Autodesk Fusion 360 part; units mm, degrees
(part 9 of 9)
extrude "Extrude4''" add sketch "Sketch1 (3)" along normal blind 2 contours A4 L3 A7 L4 L6 | A4 L2 A7 L5 L7 | A4 A5 L6 L7 | A7 A8 L6 L7 picked at (-8.5623, -94.7426) picked at (8.642, -94.7512) picked at (-12.4732, -65.0425) picked at (-12.3684, -117.2548) bodies 6 in component "Base"
extrude "Extrude5'" add sketch "Sketch1 (3)" along normal blind 1 from surface at 2 contours A4 A5 L6 L8 | A4 A7 L6 L8 | A7 A8 L6 L8 | A4 A7 L7 L9 | A4 A5 L7 L9 | A7 A8 L7 L9 | A5 L7 A9 L8 L9 | A8 A10 L8 L9 picked at (-4.204, -76.7531) picked at (-3.6307, -94.1364) picked at (-4.18, -104.3491) picked at (3.6752, -86.9585) picked at (4.2245, -76.7458) picked at (4.2486, -104.3417) picked at (-4.5123, -61.3284) picked at (5.702, -117.4496) bodies 6 7 in component "Base"
extrude "Extrude6" add 1 faces at (-0.2078, -65.36, 13) along direction (0, 0, 1) blind 4.5 on bodies 4 bodies 4 in component "slider"
component "Spur Gear 24 teeth" placed x (1, 0, 0) y (0, 1, 0) z (0, 0, 1) at (0, 0, 0)
component "Spur Gear 12 teeth" placed x (0.965926, 0.258819, 0) y (-0.258819, 0.965926, 0) z (0, 0, 1) at (0, 54, 0)
component "arm" placed x (1, 0, 0) y (0, 1, 0) z (0, 0, 1) at (0, 0, 5)
component "slider" placed x (1, 0, 0) y (0, 1, 0) z (0, 0, 1) at (0, 0, 0)
component "Base" placed x (1, 0, 0) y (0, 1, 0) z (0, 0, 1) at (0, 0, 0)
